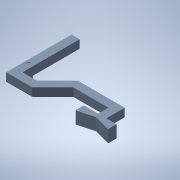
# Autodesk Inventor part: Slder43
Saved by Autodesk Inventor 2021 (Build 250183000, 183)
## iProperties
Created: 2015-03-05
Part Number: Slder43
Document SubType Name: Modeling
Designer: Administrator
Density: 1 g/cm^3
Mass: 0.20366 g
Surface Area: 4.21277 cm^2
Volume: 0.20366 cm^3
Material: Generic
Appearance: Light Steel Blue
Author: Administrator
Autodesk Inventor part; units mm, degrees
ref_plane "YZ Plane" through (0, 0, 0) normal (1, 0, 0) x (0, 1, 0)
ref_plane "XZ Plane" through (0, 0, 0) normal (0, 1, 0) x (-1, 0, 0)
ref_plane "XY Plane" through (0, 0, 0) normal (0, 0, 1) x (1, 0, 0)
sketch "Sketch8" plane through (0, 0, 0) normal (0, 0, 1) x (1, 0, 0)
  line L0 (0, 0) -> (0, 15) construction
  line L1 (0, 0) -> (5, 0) construction
  line L2 (5, 0) -> (10, 5) construction
  line L3 (10, 5) -> (20, 5) construction
  line L4 (20, 5) -> (20, 0) construction
  line L5 (21, 0) -> (21, 6)
  line L6 (21, 6) -> (9.5858, 6)
  line L7 (9.5858, 6) -> (4.5858, 1)
  line L8 (4.5858, 1) -> (1, 1)
  line L9 (1, 1) -> (1, 15)
  line L10 (19, 0) -> (19, 4)
  line L11 (19, 4) -> (10.4142, 4)
  line L12 (10.4142, 4) -> (5.4142, -1)
  line L13 (5.4142, -1) -> (-1, -1)
  line L14 (-1, -1) -> (-1, 15)
  line L15 (19, 0) -> (21, 0)
  line L16 (-1, 15) -> (1, 15)
  dimension "d49" = 15
  dimension "d50" = 5
  dimension "d51" = 45
  dimension "d52" = 5
  dimension "d53" = 20
  dimension "d54" = 5
  dimension "d55" = 1
  dimension "d56" = 1
  dimension "d62" = 0
  constraints: 34 end point, 7 perpendicular, 4 parallel, 1 vertical, 9 other
  measures "d49" distance of L0.start L0.end
  measures "d50" distance of L0.start L1.end
  measures "d51" angle of L2 L1
  measures "d52" distance between parallel lines of L3 L1
  measures "d53" distance between parallel lines of L4 L0
  measures "d54" distance of L3.end L4.end
  measures "d55" distance between parallel lines of L9 L0
  measures "d56" distance between parallel lines of L14 L0
  measures "d62" distance between parallel lines of L1 L15
extrude "Extrusion10" add sketch "Sketch8" along normal mid plane 2
sketch "Sketch9" plane through (0, 0, -1) normal (0, 0, -1) x (-1, 0, 0)
  line L0 (1, -1) -> (-5.4142, -1) projected
  line L1 (-1, 15) -> (1, 15) projected
  line L2 (-1, 1) -> (-1, 15) projected
  line L3 (0, 15) -> (0, -1) construction
  circle A0 centre (0, 3.5063) radius 0.75
  dimension "d59" = 1.5
  constraints: 2 end point, 2 point on line, 1 centre point, 1 midpoint, 1 parallel
  measures "d59" diameter of A0
extrude "Extrusion11" add sketch "Sketch9" along normal blind 1.5
sketch "Sketch10" plane through (0, 0, 1) normal (0, 0, 1) x (1, 0, 0)
  line L0 (21, 0) -> (19, 0) projected
  line L1 (19, 0) -> (19, 4) projected
  line L2 (5.4142, -1) -> (24, -1) construction
  line L3 (20, 0) -> (20, -1) construction
  line L4 (24, -1) -> (16, -1) construction
  line L5 (16, -1) -> (16, 1)
  line L6 (16, 1) -> (24, 1)
  line L7 (24, 1) -> (24, -1)
  line L8 (20, 0) -> (16.2679, -1)
  line L9 (20, 0) -> (23.7321, -1)
  line L10 (16, -1) -> (16.2679, -1)
  line L11 (23.7321, -1) -> (24, -1)
  dimension "d63" = 2
  dimension "d64" = 4
  dimension "d65" = 8
  dimension "d66" = 15
  constraints: 20 end point, 4 perpendicular, 2 parallel, 2 point on line, 1 collinear, 1 horizontal, 1 midpoint, 1 symmetric about line
  measures "d63" distance of L4.end L5.end
  measures "d64" distance between parallel lines of L7 L3
  measures "d65" distance of L5.end L6.end
  measures "d66" angle of L8 L2
extrude "Extrusion12" add sketch "Sketch10" against normal up to surface (2 mm away)
sketch "Sketch11" plane through (0, 0, 0) normal (0, 0, 1) x (1, 0, 0)
  line L0 (21, 6) -> (21, 1) projected
  line L1 (9.5858, 6) -> (21, 6) projected
  line L2 (4.5858, 1) -> (9.5858, 6) projected
  line L3 (1, 1) -> (4.5858, 1) projected
  line L4 (1, 15) -> (1, 1) projected
  line L5 (-1, 15) -> (1, 15) projected
  line L6 (-1, -1) -> (-1, 15) projected
  line L7 (5.4142, -1) -> (-1, -1) projected
  line L8 (10.4142, 4) -> (5.4142, -1) projected
  line L9 (19, 4) -> (10.4142, 4) projected
  line L10 (19, 1) -> (19, 4) projected
  line L11 (19, 1) -> (16, 1) projected
  line L12 (16, 1) -> (16, -1) projected
  line L13 (16, -1) -> (16.2679, -1) projected
  line L14 (16.2679, -1) -> (20, 0) projected
  line L15 (20, 0) -> (23.7321, -1) projected
  line L16 (23.7321, -1) -> (24, -1) projected
  line L17 (24, -1) -> (24, 1) projected
  line L18 (24, 1) -> (21, 1) projected
  line L19 (16, 1) -> (24, 1)
  constraints: 2 end point, 1 collinear
extrude "Extrusion13" add sketch "Sketch11" along normal mid plane 3 contours L18 L17 L16 L15 L14 L13 L12 L11 L19
sketch "Sketch12" plane through (0, 0, 1) normal (0, 0, 1) x (1, 0, 0)
  circle A0 centre (0, 3.5063) radius 0.75 projected
  circle A1 centre (0, 3.5063) radius 0.75 projected
  circle A2 centre (0, 3.5063) radius 0.5
  dimension "d71" = 1
  constraints: 1 centre point
  measures "d71" diameter of A2
extrude "Extrusion14" cut sketch "Sketch12" against normal blind 0.1 contours A2
body "Solid1"
